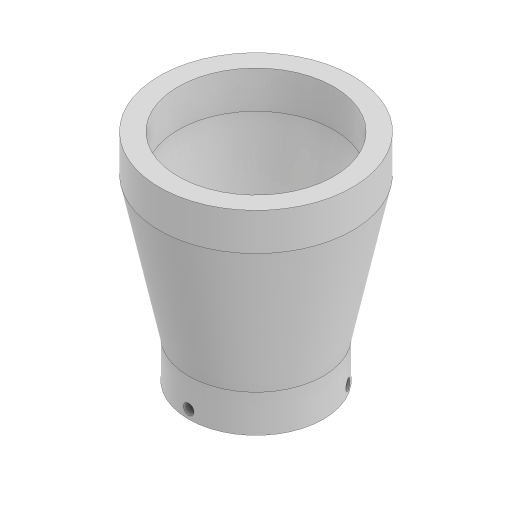
# Autodesk Inventor part: 00_Zeiss_Daheng_Adapter
Saved by Autodesk Inventor 2024.1 (Build 281209000, 209)
## iProperties
Created: 2024-04-11
Part Number: 00_Zeiss_Daheng_Adapter
Material: Generisch
Document SubType Name: Modeling
Designer: diederichbenedict
Density: 1 g/cm^3
Appearance: Vorgabe
Author: diederichbenedict
Autodesk Inventor part; units mm, degrees
ref_plane "YZ Plane" through (0, 0, 0) normal (1, 0, 0) x (0, 1, 0)
ref_plane "XZ Plane" through (0, 0, 0) normal (0, 1, 0) x (-1, 0, 0)
ref_plane "XY Plane" through (0, 0, 0) normal (0, 0, 1) x (1, 0, 0)
sketch "Skizze1" plane through (0, 0, 0) normal (1, 0, 0) x (0, 1, 0)
  line L0 (25.8, 0) -> (20.8, 0)
  line L1 (20.8, 0) -> (20.8, -10)
  line L2 (20.8, -10) -> (25.8, -10)
  line L3 (25.8, -10) -> (25.8, 0)
  line L4 (18, -57.6) -> (12, -57.6)
  line L5 (12, -57.6) -> (12, -47.6)
  line L6 (12, -47.6) -> (18, -47.6)
  line L7 (18, -47.6) -> (18, -57.6)
  line L8 (25.8, -10) -> (18, -47.6)
  line L9 (20.8, -10) -> (12, -47.6)
  line L10 (12, -57.6) -> (15, -57.6)
  line L11 (15, -57.6) -> (15, -52.6)
  line L12 (15, -52.6) -> (12, -52.6)
  line L13 (12, -52.6) -> (12, -57.6)
  line L14 (0, -70.72) -> (0, 21.12) projected
  line L15 (25.8, 0) -> (20.8, 0)
  line L16 (20.8, 0) -> (20.8, 8)
  line L17 (20.8, 8) -> (25.8, 8)
  line L18 (25.8, 8) -> (25.8, 0)
  line L19 (25.8, 0) -> (28.8, 0)
  line L20 (28.8, 0) -> (28.8, -3)
  line L21 (28.8, -3) -> (25.8, -3)
  line L22 (25.8, -3) -> (25.8, 0)
  line L23 (28.8, -3) -> (25.8, -5.6618)
  point P0 (0, 0)
  point P1 (15, -57.6)
  point P2 (15, -47.6)
  point P3 (15, -55.1)
  dimension "d0" = 5
  dimension "d1" = 10
  dimension "d2" = 25.8
  dimension "d3" = 57.6
  dimension "d4" = 10
  dimension "d5" = 6
  dimension "d6" = 12
  dimension "d7" = 5
  dimension "d8" = 15
  dimension "d16" = 8
  dimension "d17" = 3
  dimension "d18" = 3
  constraints: 46 end point, 10 parallel, 5 horizontal, 5 perpendicular, 3 midpoint, 1 point on line
  measures "d0" distance of L2.end L1.end
  measures "d1" distance of L1.end L0.end
  measures "d2" distance from line of point (0, 0) L3
  measures "d3" vertical distance of point (15, -57.6) point (0, 0)
  measures "d4" distance of point (15, -57.6) point (15, -47.6)
  measures "d5" distance between parallel lines of L5 L7
  measures "d6" horizontal distance of point (0, 0) L4.end
  measures "d7" distance of L11.end L10.end
  measures "d8" horizontal distance of point (15, -55.1) point (0, 0)
  measures "d16" distance of L15.end L16.end
  measures "d17" distance of L20.end L21.end
  measures "d18" distance of L19.end L20.end
revolve "Umdrehung1" add sketch "Skizze1" angle 360 about axis through (0, 0, -10) along (0, 0, 1) contours L3 L2 L1 L0 | L2 L8 L6 L9 | L6 L7 L4 L11 L12 L5
sketch "Skizze2" plane through (0, 0, 0) normal (0, 1, 0) x (-1, 0, 0)
  circle A0 centre (0, -55.252) radius 1.4
  point P0 (0, 0)
  dimension "d10" = 2.8
  constraints: 1 centre point
  measures "d10" diameter of A0
extrude "Extrusion1" cut sketch "Skizze2" against normal through all
pattern_circular "Runde Anordnung1" count 3 over 360 about axis through (0, 0, -52.6) along (0, 0, 1) of "Extrusion1"
